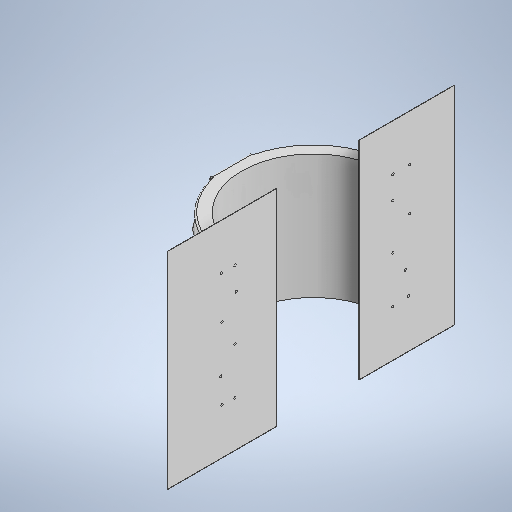
# Autodesk Inventor part: motor-mount
Saved by Autodesk Inventor 2025.2 (Build 292293000, 293)
## iProperties
Created: 2025-02-07
Part Number: motor-mount
Material: 一般
Document SubType Name: Modeling
Designer: mahhy
Density: 1 g/cm^3
Appearance: 既定
Author: mahhy
## iProperties of the stored document motor-mount_3D プリント.ipt
Created: 2025-02-10
Part Number: motor-mount_3D プリント
Material: 一般
Document SubType Name: Modeling
Designer: mahhy
Density: 1 g/cm^3
Appearance: 既定
Author: mahhy
Autodesk Inventor part; units mm, degrees
ref_plane "YZ Plane" through (0, 0, 0) normal (1, 0, 0) x (0, 1, 0)
ref_plane "XZ Plane" through (0, 0, 0) normal (0, 1, 0) x (-1, 0, 0)
ref_plane "XY Plane" through (0, 0, 0) normal (0, 0, 1) x (1, 0, 0)
sketch "スケッチ1" plane through (0, 0, 0) normal (0, 1, 0) x (-1, 0, 0)
  line L0 (0, 0) -> (60, 0)
  line L1 (60, 0) -> (60, -120)
  line L2 (60, -120) -> (0, -120)
  line L3 (0, -120) -> (0, 0)
  circle A0 centre (0, -60) radius 46
  circle A1 centre (0, -60) radius 54
  line L4 (0, -14) -> (7, -14)
  line L5 (7, -14) -> (7, 4)
  line L6 (7, 4) -> (0, 4)
  line L7 (0, 4) -> (0, -14)
  line L8 (0, -106) -> (7, -106)
  line L9 (7, -106) -> (7, -124)
  line L10 (7, -124) -> (0, -124)
  line L11 (0, -124) -> (0, -106)
  line L12 (54, -47.5) -> (46, -47.5)
  line L13 (46, -47.5) -> (46, -72.5)
  line L14 (46, -72.5) -> (54, -72.5)
  line L15 (54, -72.5) -> (54, -47.5)
  point P0 (46, -60)
  point P1 (46, -60)
  point P2 (7, -113.5444)
  point P3 (52.5333, -72.5)
  point P4 (52.5333, -47.5)
  point P5 (7, -6.4556)
  point P6 (7, 0)
  dimension "d0" = 60
  dimension "d1" = 120
  dimension "d2" = 92
  dimension "d3" = 108
  dimension "d4" = 7
  dimension "d5" = 18
  dimension "d6" = 7
  dimension "d7" = 18
  dimension "d8" = 8
  dimension "d9" = 25
  dimension "d11" = 0
  dimension "d12" = 0
  constraints: 32 end point, 8 parallel, 4 horizontal, 4 perpendicular, 3 point on circle, 2 centre point, 2 midpoint, 2 point on line, 1 coincident
  measures "d0" distance of L1.end L2.end
  measures "d1" distance of L0.end L1.end
  measures "d2" diameter of A0
  measures "d3" diameter of A1
  measures "d4" distance of L6.end L5.end
  measures "d5" distance of L5.end L4.end
  measures "d6" distance of L9.end L10.end
  measures "d7" distance of L8.end L9.end
  measures "d8" distance of L14.end L13.end
  measures "d9" distance of L13.end L12.end
  measures "d11" vertical distance of A0.centre point (46, -60)
  measures "d12" distance of point (46, -60) point (46, -60)
extrude "押し出し1" add sketch "スケッチ1" along normal blind 80 contours L7 L6 L5 L0 | L0 L5 A1 L3 | A1 L5 L4 L3 | A1 L12 L13 A0 L4 L5 | A1 L9 L2 L3 | L3 L8 L9 A1 | L12 L15 A1 | A1 L14 L13 L12 | A0 L13 L14 A1 L9 L8 | L2 L9 L10 L11 | L15 L14 A1
sketch "スケッチ2" plane through (-54, 0, -72.5) normal (-1, 0, 0) x (0, 0, 1)
  line L0 (-33.5, 0) -> (58.5, 0) projected
  line L1 (0, 0) -> (0, 80) projected
  circle A0 centre (12.5, 40) radius 12.5
  point P0 (72.5, 0)
  point P1 (12.5, 0)
  point P2 (0, 40)
  point P3 (0, 40)
  dimension "d15" = 0
  dimension "d16" = 0
  dimension "d17" = 25
  constraints: 3 midpoint, 1 centre point, 1 coincident
  measures "d15" horizontal distance of point (12.5, 0) point (12.5, 40)
  measures "d16" vertical distance of point (12.5, 40) point (0, 40)
  measures "d17" diameter of A0
extrude "押し出し2" add sketch "スケッチ2" along normal blind 1
sketch "スケッチ3" plane through (-55, 40, -60) normal (-1, 0, 0) x (0, 0, 1)
  circle A0 centre (0, 0) radius 8.5
  point P0 (60, -40)
  dimension "d20" = 17
  constraints: 1 centre point
  measures "d20" diameter of A0
extrude "押し出し3" add sketch "スケッチ3" along normal blind 15
sketch "スケッチ4" plane through (-7, 0, -124) normal (-1, 0, 0) x (0, 0, 1)
  line L0 (0, 80) -> (10.4556, 80) projected
  line L1 (0, 0) -> (10.4556, 0) projected
  line L2 (117.5444, 80) -> (128, 80) projected
  line L3 (117.5444, 0) -> (124, 0) projected
  point P0 (5.2278, 70)
  point P1 (5.2278, 10)
  point P2 (122.7722, 10)
  point P3 (5.2278, 80)
  point P4 (5.2278, 0)
  point P5 (120.7722, 0)
  point P6 (122.7722, 70)
  point P7 (122.7722, 80)
  dimension "d23" = 0
  dimension "d24" = 10
  dimension "d25" = 0
  dimension "d26" = 10
  dimension "d28" = 10
  dimension "d36" = 0
  dimension "d37" = 10
  constraints: 4 midpoint
  measures "d23" horizontal distance of point (5.228, 80) point (5.228, 70)
  measures "d24" distance from line of L0 point (5.228, 70)
  measures "d25" horizontal distance of point (5.228, 0) point (5.228, 10)
  measures "d26" distance from line of L1 point (5.228, 10)
  measures "d28" vertical distance of point (120.772, 0) point (122.772, 10)
  measures "d36" horizontal distance of point (122.772, 80) point (122.772, 70)
  measures "d37" distance from line of L2 point (122.772, 70)
hole "穴1" at (-7, 70, -118.7722) at (-7, 10, -118.7722) at (-7, 10, -1.2278) at (-7, 70, -1.2278) direction (1, 0, 0) diameter 4.2 end through all
fillet "フィレット1" radius 1 12 edges at (-3.5, 80, -124) (-3.5, 80, 4) (-7, 80, -1.2278) (-7, 80, -118.7722) (-36.1554, 80, -100.1097) (-36.1554, 80, -19.8903) (-7, 40, 4) (-36.1554, 0, -19.8903) (-3.5, 0, 4) (-36.1554, 0, -100.1097) (-3.5, 0, -124) (-7, 0, -118.7722)
fillet "フィレット2" radius 2 2 edges at (-54, 80, -60) (-54, 0, -60)
fillet "フィレット3" radius 1 2 edges at (-55, 40, -72.5) (-70, 40, -68.5)
fillet "フィレット4" radius 1 6 edges at (-6.669, 79.7433, -113.253) (-6.669, 0.2567, -113.253) (-7, 40, -113.5444) (-6.669, 79.7433, -6.747) (-7, 0.2921, -6.7518) (-7, 40, -6.4556)
sketch "スケッチ7" plane through (0, 0, -106) normal (1, 0, 0) x (0, 0, -1)
  circle A0 centre (-106, 76.3783) radius 0.75
  circle A1 centre (-97.1776, 2.7289) radius 0.75
  circle A2 centre (14.4403, 3.4789) radius 0.75
  line L0 (7.4257, 1) -> (7.4257, 79) projected
  circle A3 centre (-96.4276, 61.3872) radius 0.75
  circle A4 centre (-97.1776, 32.6177) radius 0.75
  circle A5 centre (-106.2974, 19.12) radius 0.75
  circle A6 centre (4.385, 32.6177) radius 0.75
  circle A7 centre (15.1903, 49.0782) radius 0.75
  circle A8 centre (15.1903, 76.3783) radius 0.75
  circle A9 centre (4.385, 2.7289) radius 0.75
  circle A10 centre (12.3425, 19.12) radius 0.75
  circle A11 centre (4.385, 61.7398) radius 0.75
  circle A12 centre (4.385, 76.3783) radius 0.75
  circle A13 centre (-97.1776, 76.3783) radius 0.75
  circle A14 centre (-105.5474, 49.0782) radius 0.75
  circle A15 centre (-105.5474, 2.8818) radius 0.75
  point P0 (-106, 0)
  dimension "d51" = 1.5
  dimension "d52" = 1.5
  dimension "d53" = 1.5
  dimension "d57" = 1.5
  dimension "d58" = 1.5
  dimension "d59" = 1.5
  dimension "d60" = 1.5
  dimension "d61" = 1.5
  dimension "d62" = 1.5
  dimension "d63" = 1.5
  dimension "d64" = 1.5
  dimension "d65" = 1.5
  dimension "d66" = 1.5
  dimension "d67" = 1.5
  dimension "d68" = 1.5
  dimension "d69" = 1.5
  constraints: 16 centre point
  measures "d51" diameter of A0
  measures "d52" diameter of A1
  measures "d53" diameter of A2
  measures "d57" diameter of A3
  measures "d58" diameter of A4
  measures "d59" diameter of A5
  measures "d60" diameter of A6
  measures "d61" diameter of A7
  measures "d62" diameter of A8
  measures "d63" diameter of A9
  measures "d64" diameter of A10
  measures "d65" diameter of A11
  measures "d66" diameter of A12
  measures "d67" diameter of A13
  measures "d68" diameter of A14
  measures "d69" diameter of A15
extrude "押し出し6" add sketch "スケッチ7" along normal blind 0.8
sketch "スケッチ8" plane through (0.8, 61.3872, -9.5724) normal (1, 0, 0) x (0, 0, -1)
  line L0 (-44.228, 44.6054) -> (25.6462, 44.6054)
  line L1 (25.6462, 44.6054) -> (25.6462, -87.9969)
  line L2 (25.6462, -87.9969) -> (-44.228, -87.9969)
  line L3 (-44.228, -87.9969) -> (-44.228, 44.6054)
  line L4 (78.8459, 44.9372) -> (140.3829, 44.9372)
  line L5 (140.3829, 44.9372) -> (140.3829, -88.6081)
  line L6 (140.3829, -88.6081) -> (78.8459, -88.6081)
  line L7 (78.8459, -88.6081) -> (78.8459, 44.9372)
  point P0 (-9.5724, -61.3872)
  constraints: 16 end point, 4 parallel, 2 horizontal, 2 perpendicular
extrude "押し出し7" add sketch "スケッチ8" along normal blind 0.2
